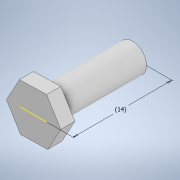
# Autodesk Inventor part: nut1
Saved by Autodesk Inventor 2022 (Build 260153070, 153G)
## iProperties
Created: 2021-07-09
Part Number: nut1
Material: Generic
Document SubType Name: Modeling
Designer: 91852
Density: 1 g/cm^3
Appearance: Default
Author: 91852
Autodesk Inventor part; units mm, degrees
ref_plane "YZ Plane" through (0, 0, 0) normal (1, 0, 0) x (0, 1, 0)
ref_plane "XZ Plane" through (0, 0, 0) normal (0, 1, 0) x (-1, 0, 0)
ref_plane "XY Plane" through (0, 0, 0) normal (0, 0, 1) x (1, 0, 0)
sketch "Sketch1" plane through (0, 0, 0) normal (0, 0, 1) x (1, 0, 0)
  circle A0 centre (0, 0) radius 2
  dimension "d0" = 4
  constraints: 1 centre point, 1 coincident
  measures "d0" diameter of A0
extrude "Extrusion1" add sketch "Sketch1" along normal blind 12
sketch "Sketch2" plane through (0, 0, 12) normal (0, 0, 1) x (1, 0, 0)
  line L0 (2, -3.2858) -> (-1.8456, -3.375)
  line L1 (-1.8456, -3.375) -> (-3.8456, -0.0891)
  line L2 (-3.8456, -0.0891) -> (-2, 3.2858)
  line L3 (-2, 3.2858) -> (1.8456, 3.375)
  line L4 (1.8456, 3.375) -> (3.8456, 0.0891)
  line L5 (3.8456, 0.0891) -> (2, -3.2858)
  point P0 (0, 0)
  point P1 (0, 0)
  constraints: 12 end point, 1 coincident, 13 other
extrude "Extrusion2" add sketch "Sketch2" along normal blind 2
sketch "Sketch3" plane through (0, 0, 0) normal (0, 1, 0) x (-1, 0, 0)
  line L0 (-1.8456, 14) -> (2, 14) projected
  line L1 (2, 0) -> (-2, 0) projected
  point P0 (0, 0)
  dimension "d5" = 14
  measures "d5" distance between parallel lines of L0 L1
body "Solid1"
